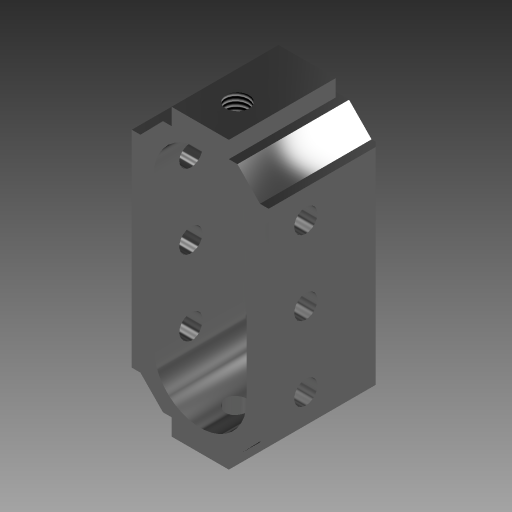
# Autodesk Inventor part: REVLIFT-MAXTube Blocks
Saved by Autodesk Inventor 2023 (Build 270158000, 158)
## iProperties
Created: 2022-12-30
Part Number: REVLIFT-MAXTube Blocks
Material: Aluminum 6061
Document SubType Name: Modeling
Designer: Max Boord
Mass: 24.7455 g
Surface Area: 63.4102 cm^2
Volume: 9.165 cm^3
Density: 2.7 g/cm^3
Appearance: Glazed - Black
Mass: 31.6626 g
Surface Area: 60.3795 cm^2
Volume: 11.7269 cm^3
Author: Max Boord
Mass: 14.9913 g
Surface Area: 30.4821 cm^2
Volume: 5.55233 cm^3
Mass: 27.7622 g
Surface Area: 58.342 cm^2
Volume: 10.2823 cm^3
Autodesk Inventor part; units mm, degrees
ref_plane "YZ Plane" through (0, 0, 0) normal (1, 0, 0) x (0, 1, 0)
ref_plane "XZ Plane" through (0, 0, 0) normal (0, 1, 0) x (-1, 0, 0)
ref_plane "XY Plane" through (0, 0, 0) normal (0, 0, 1) x (1, 0, 0)
sketch "Sketch1" plane through (0, 0, 0) normal (0, 0, 1) x (1, 0, 0)
  line L0 (12.7, 25.4) -> (-12.7, 25.4) construction
  line L1 (-12.7, 25.4) -> (-12.7, -25.4) construction
  line L2 (-12.7, -25.4) -> (12.7, -25.4) construction
  line L3 (12.7, -25.4) -> (12.7, 25.4) construction
  line L4 (12.7, 25.4) -> (-12.7, -25.4) construction
  line L5 (-12.7, 25.4) -> (12.7, -25.4) construction
  line L6 (-12.7, 0) -> (12.7, 0) construction
  line L7 (0, 25.4) -> (0, -25.4) construction
  line L8 (4.8895, 24.384) -> (4.8895, 21.5273)
  line L9 (4.8895, -24.384) -> (4.8895, -21.5273)
  line L10 (-11.684, 17.5895) -> (-12.7, 17.5895)
  line L11 (12.7, 17.5895) -> (11.684, 17.5895)
  line L12 (-11.684, -17.5895) -> (-12.7, -17.5895)
  line L13 (12.7, -17.5895) -> (11.684, -17.5895)
  line L14 (-11.684, -24.384) -> (-11.684, 24.384)
  line L15 (-11.684, 24.384) -> (11.684, 24.384)
  line L16 (11.684, 24.384) -> (11.684, -24.384)
  line L17 (11.684, -24.384) -> (-11.684, -24.384)
  line L18 (10.2108, -17.5895) -> (6.3627, -21.5273)
  line L19 (10.2108, 17.5895) -> (6.3627, 21.5273)
  line L20 (6.3627, -21.5273) -> (4.8895, -21.5273)
  line L21 (4.8895, 21.5273) -> (6.3627, 21.5273)
  line L22 (10.2108, -17.5895) -> (11.684, -17.5895)
  line L23 (11.684, 17.5895) -> (10.2108, 17.5895)
  line L24 (-4.8895, 24.384) -> (-4.8895, 21.5273)
  line L25 (-4.8895, -24.384) -> (-4.8895, -21.5273)
  line L26 (-10.2108, -17.5895) -> (-6.3627, -21.5273)
  line L27 (-10.2108, 17.5895) -> (-6.3627, 21.5273)
  line L28 (-6.3627, -21.5273) -> (-4.8895, -21.5273)
  line L29 (-4.8895, 21.5273) -> (-6.3627, 21.5273)
  line L30 (-10.2108, -17.5895) -> (-11.684, -17.5895)
  line L31 (-11.684, 17.5895) -> (-10.2108, 17.5895)
  point P0 (0, 0)
  point P1 (0, 0)
  point P2 (4.8895, 12.7)
  point P3 (-4.8895, -12.7)
  point P4 (4.8895, -12.7)
  point P5 (4.8895, 11.684)
  point P6 (-11.684, 4.8895)
  point P7 (-11.684, -4.8895)
  point P8 (9.525, -4.8895)
  point P9 (9.525, 4.8895)
  point P10 (4.8895, -11.684)
  point P11 (11.684, 0)
  point P12 (0, 0)
  point P13 (0, -24.384)
  point P14 (-4.8895, 12.7)
  point P15 (-4.8895, -12.7)
  point P16 (-11.684, 0)
  point P17 (-9.2737, 17.5895)
  point P18 (-9.2737, -17.5895)
  dimension "d0" = 25.4
  dimension "d1" = 50.8
  dimension "d4" = 1.016
  dimension "d7" = 35.179
  dimension "d11" = 1.016
  dimension "d46" = 44.34
  dimension "d48" = 1.4732
  dimension "d49" = 9.779
  constraints: 64 end point, 15 symmetric about line, 10 midpoint, 9 point on line, 5 horizontal, 4 parallel, 3 collinear, 3 equal length, 3 perpendicular, 1 horizontal alignment, 1 vertical, 1 vertical alignment, 1 other
  measures "d0" distance of L2.end L1.end
  measures "d1" distance of L1.end L0.end
  measures "d4" distance between parallel lines of L1 L14
  measures "d7" distance between parallel lines of L10 L12
  measures "d11" distance between parallel lines of L0 L15
  measures "d46" angle of L16 L18
  measures "d48" distance from line of L9 L18.end
  measures "d49" distance between parallel lines of L8 L24
extrude "Extrusion1" add sketch "Sketch1" along normal blind 6.35 and the other way blind 12.7 contours L8 L21 L19 L23 L16 L22 L18 L20 L9 L17 L25 L28 L26 L30 L14 L31 L27 L29 L24 L15
sketch "Sketch2" plane through (0, 0, 6.35) normal (0, 0, 1) x (1, 0, 0)
  point P0 (0, 0)
hole "Hole1" at (0, 0, 6.35) direction (0, 0, -1) diameter 3.9624 end through all thread size "10-32 UNF" class "2B" standard "ANSI Unified Screw Threads"
pattern_linear "Rectangular Pattern1" count 3 spacing 12.7 along (0, 1, 0) of "Hole1" first direction both ways yes
pattern_circular "Circular Pattern1" count 3 over 180 about axis through (0, -10, 0) along (0, 1, 0) of "Hole1", "Rectangular Pattern1" both ways yes
sketch "Sketch3" plane through (-4.8895, 24.384, 6.35) normal (0, 1, 0) x (1, 0, 0)
  point P0 (4.8895, 6.35)
hole "Hole2" at (0, 24.384, 0) direction (0, -1, 0) diameter 3.9624 end through all thread size "10-32 UNF" class "2B" standard "ANSI Unified Screw Threads"
chamfer "Chamfer1" distance 0.7937 angle 45 4 edges at (0, 24.384, -12.7) (4.8895, 22.9556, -12.7) (11.684, 0, -12.7) (-11.684, 0, -12.7)
sketch "Sketch4" plane through (0, 0, 6.35) normal (0, 0, 1) x (1, 0, 0)
  line L0 (0, 12.7) -> (0, -12.7) construction
  line L1 (7.9375, 12.7) -> (7.9375, -12.7)
  line L2 (-7.9375, -12.7) -> (-7.9375, 12.7)
  arc A0 (7.9375, 12.7) -> (-7.9375, 12.7) centre (0, 12.7) ccw
  arc A1 (-7.9375, -12.7) -> (7.9375, -12.7) centre (0, -12.7) ccw
  point P0 (0, 0)
  point P1 (0, -12.7)
  dimension "d39" = 15.875
  dimension "d43" = 25.4
  constraints: 8 end point, 4 point on circle, 4 tangent, 2 centre point, 1 midpoint, 1 parallel, 1 vertical
  measures "d39" distance between parallel lines of L1 L2
  measures "d43" distance of L0.start L0.end
extrude "Extrusion2" cut sketch "Sketch4" against normal blind 15.875
fillet "Fillet1" radius 0.7937 4 edges at (7.9375, 0, -9.525) (0, -20.6375, -9.525) (-7.9375, 0, -9.525) (0, 20.6375, -9.525)
body "Solid1"
